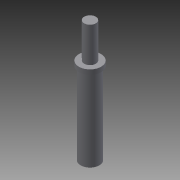
# Autodesk Inventor part: hobbing_jig_shaft
Saved by Autodesk Inventor 2014 (Build 180170000, 170)
## iProperties
Created: 2014-01-05
Part Number: hobbing_jig_shaft
Material: Generic
Document SubType Name: Modeling
Designer: caleb
Density: 1 g/cm^3
Appearance: Default
Author: caleb
Autodesk Inventor part; units mm, degrees
ref_plane "YZ Plane" through (0, 0, 0) normal (1, 0, 0) x (0, 1, 0)
ref_plane "XZ Plane" through (0, 0, 0) normal (0, 1, 0) x (-1, 0, 0)
ref_plane "XY Plane" through (0, 0, 0) normal (0, 0, 1) x (1, 0, 0)
sketch "Sketch1" plane through (0, 0, 0) normal (1, 0, 0) x (0, 1, 0)
  line L0 (0, 0) -> (4, 0)
  line L1 (4, 0) -> (4, 35)
  line L2 (4, 35) -> (4.75, 35)
  line L3 (4.75, 35) -> (4.75, 37)
  line L4 (4.75, 37) -> (2.5, 37)
  line L5 (2.5, 37) -> (2.5, 52)
  line L6 (2.5, 52) -> (0, 52)
  line L7 (0, 52) -> (0, 0)
  dimension "d0" = 4
  dimension "d1" = 4.75
  dimension "d2" = 35
  dimension "d3" = 2
  dimension "d4" = 15
  dimension "d5" = 2.5
  constraints: 16 end point, 6 parallel, 1 horizontal, 1 perpendicular
  measures "d0" distance of L0.start L0.end
  measures "d1" horizontal distance of L0.start L2.end
  measures "d2" distance of L0.end L1.end
  measures "d3" distance of L2.end L3.end
  measures "d4" distance of L4.end L5.end
  measures "d5" distance of L5.end L6.end
revolve "Revolution1" add sketch "Sketch1" angle 360 about axis through (0, 0, 52) along (0, 0, -1)
sketch "Sketch2" plane through (0, 0, 0) normal (0, 0, -1) x (-1, 0, 0)
  circle A0 centre (0, 0) radius 4 construction
  circle A1 centre (0, 0) radius 3.9688
  dimension "d12" = 7.9375
  constraints: 1 centre point, 1 coincident
  measures "d12" diameter of A1
body "Solid1"
